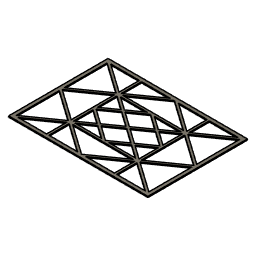
platform v3 (Autodesk Fusion 360 design; units mm, degrees)
Autodesk Fusion 360 part; units mm, degrees
sketch "Sketch1" plane through (0, 0, 0) normal (0, 1, 0) x (1, 0, 0)
  line L0 (178.39, 125.95) -> (-178.39, 125.95)
  line L1 (-178.39, 125.95) -> (-178.39, -125.95)
  line L2 (-178.39, -125.95) -> (178.39, -125.95)
  line L3 (178.39, -125.95) -> (178.39, 125.95)
  line L4 (178.39, 125.95) -> (-178.39, -125.95) construction
  line L5 (-178.39, 125.95) -> (178.39, -125.95) construction
  line L6 (-178.39, 0) -> (0, 125.95) construction
  line L7 (0, 125.95) -> (178.39, 0) construction
  line L8 (178.39, 0) -> (0, -125.95) construction
  line L9 (-178.39, 0) -> (0, -125.95) construction
  line L10 (-89.195, -62.975) -> (89.195, -62.975) construction
  line L11 (-89.195, 62.975) -> (89.195, 62.975) construction
  line L12 (89.195, 62.975) -> (89.195, -62.975) construction
  line L13 (-89.195, -62.975) -> (-89.195, 62.975) construction
  line L14 (-89.195, 0) -> (0, 62.975) construction
  line L15 (0, 62.975) -> (89.195, 0) construction
  line L16 (89.195, 0) -> (0, -62.975) construction
  line L17 (-89.195, 0) -> (0, -62.975) construction
  line L18 (-89.195, -62.975) -> (-89.195, -125.95) construction
  line L19 (89.195, -62.975) -> (89.195, -125.95) construction
  line L20 (89.195, 62.975) -> (89.195, 125.95) construction
  line L21 (-89.195, 62.975) -> (-89.195, 125.95) construction
  line L22 (-178.39, 125.95) -> (-89.195, 62.975)
  line L23 (-89.195, 62.975) -> (-90.9253, 60.5243)
  line L24 (-90.9253, 60.5243) -> (-180.1203, 123.4993)
  line L25 (-180.1203, 123.4993) -> (-178.39, 125.95)
  line L26 (-87.4647, 65.4257) -> (-176.6597, 128.4007)
  line L27 (-89.195, 62.975) -> (-87.4647, 65.4257)
  line L28 (-176.6597, 128.4007) -> (-178.39, 125.95)
  line L29 (-89.195, 125.95) -> (-89.195, 62.975)
  line L30 (-89.195, 62.975) -> (-92.195, 62.975)
  line L31 (-92.195, 62.975) -> (-92.195, 125.95)
  line L32 (-92.195, 125.95) -> (-89.195, 125.95)
  line L33 (-86.195, 62.975) -> (-86.195, 125.95)
  line L34 (-89.195, 62.975) -> (-86.195, 62.975)
  line L35 (-178.39, 0) -> (-89.195, 62.975)
  line L36 (-89.195, 62.975) -> (-90.9253, 65.4257)
  line L37 (-90.9253, 65.4257) -> (-180.1203, 2.4507)
  line L38 (-180.1203, 2.4507) -> (-178.39, 0)
  line L39 (-87.4647, 60.5243) -> (-176.6597, -2.4507)
  line L40 (-89.195, 62.975) -> (-87.4647, 60.5243)
  line L41 (-89.195, 62.975) -> (-89.195, 0)
  line L42 (-89.195, 0) -> (-92.195, 0)
  line L43 (-92.195, 0) -> (-92.195, 62.975)
  line L44 (-92.195, 62.975) -> (-89.195, 62.975)
  line L45 (-86.195, 0) -> (-86.195, 62.975)
  line L46 (-89.195, 0) -> (-86.195, 0)
  line L47 (-89.195, 0) -> (0, 62.975)
  line L48 (0, 62.975) -> (1.7303, 60.5243)
  line L49 (1.7303, 60.5243) -> (-87.4647, -2.4507)
  line L50 (-87.4647, -2.4507) -> (-89.195, 0)
  line L51 (0, 62.975) -> (-1.7303, 65.4257)
  line L52 (-1.7303, 65.4257) -> (-90.9253, 2.4507)
  line L53 (178.39, -125.95) -> (-89.195, 62.975)
  line L54 (-89.195, 62.975) -> (-87.4647, 65.4257)
  line L55 (-87.4647, 65.4257) -> (180.1203, -123.4993)
  line L56 (180.1203, -123.4993) -> (178.39, -125.95)
  line L57 (-90.9253, 60.5243) -> (176.6597, -128.4007)
  line L58 (0, 125.95) -> (-89.195, 62.975)
  line L59 (-89.195, 62.975) -> (-87.4647, 60.5243)
  line L60 (-87.4647, 60.5243) -> (1.7303, 123.4993)
  line L61 (1.7303, 123.4993) -> (0, 125.95)
  line L62 (-90.9253, 65.4257) -> (-1.7303, 128.4007)
  line L63 (-89.195, 62.975) -> (89.195, 62.975)
  line L64 (89.195, 62.975) -> (89.195, 65.975)
  line L65 (89.195, 65.975) -> (-89.195, 65.975)
  line L66 (-89.195, 65.975) -> (-89.195, 62.975)
  line L67 (89.195, 59.975) -> (-89.195, 59.975)
  line L68 (0, 62.975) -> (89.195, 0)
  line L69 (89.195, 0) -> (90.9253, 2.4507)
  line L70 (90.9253, 2.4507) -> (1.7303, 65.4257)
  line L71 (1.7303, 65.4257) -> (0, 62.975)
  line L72 (87.4647, -2.4507) -> (-1.7303, 60.5243)
  line L73 (-178.39, -125.95) -> (178.39, 125.95)
  line L74 (178.39, 125.95) -> (176.6597, 128.4007)
  line L75 (176.6597, 128.4007) -> (-180.1203, -123.4993)
  line L76 (-180.1203, -123.4993) -> (-178.39, -125.95)
  line L77 (180.1203, 123.4993) -> (-176.6597, -128.4007)
  line L78 (-89.195, -125.95) -> (-89.195, 0)
  line L79 (-89.195, 0) -> (-92.195, 0)
  line L80 (-92.195, 0) -> (-92.195, -125.95)
  line L81 (-92.195, -125.95) -> (-89.195, -125.95)
  line L82 (-86.195, 0) -> (-86.195, -125.95)
  line L83 (-178.39, 0) -> (0, -125.95)
  line L84 (0, -125.95) -> (1.7303, -123.4993)
  line L85 (1.7303, -123.4993) -> (-176.6597, 2.4507)
  line L86 (-176.6597, 2.4507) -> (-178.39, 0)
  line L87 (-1.7303, -128.4007) -> (-180.1203, -2.4507)
  line L88 (0, -62.975) -> (-89.195, 0)
  line L89 (-89.195, 0) -> (-87.4647, 2.4507)
  line L90 (-87.4647, 2.4507) -> (1.7303, -60.5243)
  line L91 (1.7303, -60.5243) -> (0, -62.975)
  line L92 (-90.9253, -2.4507) -> (-1.7303, -65.4257)
  line L93 (178.39, 0) -> (0, -125.95)
  line L94 (0, -125.95) -> (-1.7303, -123.4993)
  line L95 (-1.7303, -123.4993) -> (176.6597, 2.4507)
  line L96 (176.6597, 2.4507) -> (178.39, 0)
  line L97 (1.7303, -128.4007) -> (180.1203, -2.4507)
  line L98 (0, 125.95) -> (178.39, 0)
  line L99 (178.39, 0) -> (180.1203, 2.4507)
  line L100 (180.1203, 2.4507) -> (1.7303, 128.4007)
  line L101 (1.7303, 128.4007) -> (0, 125.95)
  line L102 (176.6597, -2.4507) -> (-1.7303, 123.4993)
  line L103 (89.195, 125.95) -> (89.195, -125.95)
  line L104 (89.195, -125.95) -> (92.195, -125.95)
  line L105 (92.195, -125.95) -> (92.195, 125.95)
  line L106 (92.195, 125.95) -> (89.195, 125.95)
  line L107 (86.195, -125.95) -> (86.195, 125.95)
  line L108 (0, -62.975) -> (89.195, 0)
  line L109 (89.195, 0) -> (87.4647, 2.4507)
  line L110 (87.4647, 2.4507) -> (-1.7303, -60.5243)
  line L111 (-1.7303, -60.5243) -> (0, -62.975)
  line L112 (90.9253, -2.4507) -> (1.7303, -65.4257)
  line L113 (-89.195, -62.975) -> (89.195, -62.975)
  line L114 (89.195, -62.975) -> (89.195, -59.975)
  line L115 (89.195, -59.975) -> (-89.195, -59.975)
  line L116 (-89.195, -59.975) -> (-89.195, -62.975)
  line L117 (89.195, -65.975) -> (-89.195, -65.975)
  line L118 (-178.39, 125.95) -> (-174.39, 125.95)
  line L119 (-174.39, 125.95) -> (-174.39, -126.4932)
  line L120 (-174.39, -126.4932) -> (-178.39, -126.4932)
  line L121 (-178.39, -126.4932) -> (-178.39, 125.95)
  line L122 (-178.39, -125.95) -> (178.39, -125.95)
  line L123 (178.39, -125.95) -> (178.39, -121.95)
  line L124 (178.39, -121.95) -> (-178.39, -121.95)
  line L125 (-178.39, -121.95) -> (-178.39, -125.95)
  line L126 (178.39, 125.95) -> (174.39, 125.95)
  line L127 (174.39, 125.95) -> (174.39, -125.95)
  line L128 (174.39, -125.95) -> (178.39, -125.95)
  line L129 (178.39, -125.95) -> (178.39, 125.95)
  line L130 (178.39, 125.95) -> (-178.39, 125.95)
  line L131 (-178.39, 125.95) -> (-178.39, 121.95)
  line L132 (-178.39, 121.95) -> (178.39, 121.95)
  line L133 (178.39, 121.95) -> (178.39, 125.95)
  line L134 (183.39, 130.95) -> (-183.39, 130.95)
  line L135 (-183.39, 130.95) -> (-183.39, -130.95)
  line L136 (-183.39, -130.95) -> (183.39, -130.95)
  line L137 (183.39, -130.95) -> (183.39, 130.95)
  line L138 (183.39, 130.95) -> (-183.39, -130.95) construction
  line L139 (-183.39, 130.95) -> (183.39, -130.95) construction
  line L140 (0, 130.95) -> (0, 125.95) construction
  line L141 (-183.39, 66.313) -> (-178.39, 66.313) construction
  dimension "d1" = 356.78
  dimension "d2" = 251.9
  dimension "d3" = 3
  dimension "d4" = 3
  dimension "d5" = 3
  dimension "d6" = 3
  dimension "d7" = 3
  dimension "d8" = 3
  dimension "d9" = 3
  dimension "d10" = 3
  dimension "d11" = 3
  dimension "d12" = 3
  dimension "d13" = 3
  dimension "d14" = 3
  dimension "d15" = 3
  dimension "d16" = 3
  dimension "d17" = 3
  dimension "d18" = 3
  dimension "d19" = 3
  dimension "d20" = 3
  dimension "d21" = 4
  dimension "d22" = 4
  dimension "d23" = 4
  dimension "d24" = 4
  dimension "d27" = 5
  constraint horizontal L0
  constraint perpendicular L0 L1
  constraint parallel L0 L2
  constraint parallel L1 L3
  constraint coincident L4 origin
  constraint coincident L5 origin
  constraint midpoint L1 L6.start
  constraint midpoint L0 L6.end
  constraint midpoint L3 L7.end
  constraint midpoint L2 L8.end
  constraint midpoint L9 L10.start
  constraint midpoint L8 L10.end
  constraint midpoint L6 L11.start
  constraint midpoint L7 L11.end
  constraint midpoint L13 L14.start
  constraint midpoint L11 L14.end
  constraint midpoint L12 L15.end
  constraint midpoint L10 L16.end
  constraint coincident L2 L18.end
  constraint perpendicular L2 L18
  constraint coincident L2 L19.end
  constraint perpendicular L2 L19
  constraint coincident L0 L20.end
  constraint perpendicular L0 L20
  constraint coincident L0 L21.end
  constraint perpendicular L0 L21
  constraint perpendicular L22 L23
  constraint parallel L22 L24
  constraint parallel L23 L25
  constraint symmetric L0.end L5 L1.start
  constraint symmetric L5 L11.start L13.end
  constraint symmetric L5 L23.end L26.start
  constraint symmetric L5 L24.end L26.end
  constraint perpendicular L29 L30
  constraint parallel L29 L31
  constraint parallel L30 L32
  constraint symmetric L21 L11.start L13.end
  constraint symmetric L21 L30.end L33.start
  constraint symmetric L21 L31.end L33.end
  constraint perpendicular L35 L36
  constraint parallel L35 L37
  constraint parallel L36 L38
  constraint symmetric L6 L11.start L13.end
  constraint symmetric L6 L36.end L39.start
  constraint symmetric L6 L37.end L39.end
  constraint perpendicular L41 L42
  constraint parallel L41 L43
  constraint parallel L42 L44
  constraint symmetric L14.start L41 L17.start
  constraint symmetric L42.end L41 L45.start
  constraint symmetric L30.end L41 L33.start
  constraint perpendicular L47 L48
  constraint parallel L47 L49
  constraint parallel L48 L50
  constraint symmetric L15.start L14 L47.end
  constraint symmetric L14 L48.end L51.end
  constraint symmetric L14 L49.end L52.end
  constraint perpendicular L53 L54
  constraint parallel L53 L55
  constraint parallel L54 L56
  constraint symmetric L26.start L53 L23.end
  constraint symmetric L55.end L53 L57.end
  constraint perpendicular L58 L59
  constraint parallel L58 L60
  constraint parallel L59 L61
  constraint symmetric L39.start L58 L36.end
  constraint symmetric L60.end L58 L62.end
  constraint perpendicular L63 L64
  constraint parallel L63 L65
  constraint parallel L64 L66
  constraint symmetric L64.end L63 L67.start
  constraint symmetric L65.end L63 L67.end
  constraint perpendicular L68 L69
  constraint parallel L68 L70
  constraint parallel L69 L71
  constraint symmetric L15 L69.end L72.start
  constraint symmetric L15 L70.end L72.end
  constraint perpendicular L73 L74
  constraint parallel L73 L75
  constraint parallel L74 L76
  constraint symmetric L4 L74.end L77.start
  constraint symmetric L4 L75.end L77.end
  constraint perpendicular L78 L79
  constraint parallel L78 L80
  constraint parallel L79 L81
  constraint symmetric L13 L42.end L45.start
  constraint symmetric L13 L80.end L82.end
  constraint perpendicular L83 L84
  constraint parallel L83 L85
  constraint parallel L84 L86
  constraint symmetric L9 L84.end L87.start
  constraint symmetric L9 L85.end L87.end
  constraint perpendicular L88 L89
  constraint parallel L88 L90
  constraint parallel L89 L91
  constraint symmetric L89.end L88 L92.start
  constraint symmetric L90.end L88 L92.end
  constraint perpendicular L93 L94
  constraint parallel L93 L95
  constraint parallel L94 L96
  constraint symmetric L8 L94.end L97.start
  constraint symmetric L8 L95.end L97.end
  constraint perpendicular L98 L99
  constraint parallel L98 L100
  constraint parallel L99 L101
  constraint symmetric L99.end L98 L102.start
  constraint symmetric L100.end L98 L102.end
  constraint perpendicular L103 L104
  constraint parallel L103 L105
  constraint parallel L104 L106
  constraint symmetric L19 L104.end L107.start
  constraint symmetric L19 L105.end L107.end
  constraint perpendicular L108 L109
  constraint parallel L108 L110
  constraint parallel L109 L111
  constraint symmetric L16 L109.end L112.start
  constraint symmetric L16 L110.end L112.end
  constraint perpendicular L113 L114
  constraint parallel L113 L115
  constraint parallel L114 L116
  constraint symmetric L10 L114.end L117.start
  constraint symmetric L10 L115.end L117.end
  constraint horizontal L118
  constraint vertical L119
  constraint horizontal L120
  constraint vertical L121
  constraint horizontal L122
  constraint vertical L123
  constraint horizontal L124
  constraint vertical L125
  constraint horizontal L126
  constraint vertical L127
  constraint horizontal L128
  constraint vertical L129
  constraint coincident L122 L127.end
  constraint horizontal L130
  constraint vertical L131
  constraint horizontal L132
  constraint vertical L133
  constraint horizontal L134
  constraint perpendicular L134 L135
  constraint parallel L134 L136
  constraint parallel L135 L137
  constraint coincident L138 origin
  constraint coincident L139 origin
  constraint midpoint L134 L140.start
  constraint coincident L135 L141.start
  constraint coincident L121 L141.end
  constraint perpendicular L121 L141
  constraint equal L140 L141
  measures "d1" distance of L0.start L0.end
  measures "d2" distance of L0.start L2.end
  measures "d3" distance of L0.end L24.end
  measures "d4" distance of L21.end L31.end
  measures "d5" distance of L6.start L37.end
  measures "d6" distance of L11.start L30.end
  measures "d7" distance of L14.start L49.end
  measures "d8" distance of L2.end L55.end
  measures "d9" distance of L6.end L60.end
  measures "d10" distance of L11.start L65.end
  measures "d11" distance of L14.end L70.end
  measures "d12" distance of L1.end L75.end
  measures "d13" distance of L18.end L80.end
  measures "d14" distance of L6.start L85.end
  measures "d15" distance of L16.end L90.end
  measures "d16" distance of L7.end L95.end
  measures "d17" distance of L6.end L100.end
  measures "d18" distance of L20.end L105.end
  measures "d19" distance of L16.end L110.end
  measures "d20" distance of L10.start L115.end
  measures "d21" distance of L0.end L118.end
  measures "d22" distance of L1.end L124.end
  measures "d23" distance of L0.start L126.end
  measures "d24" distance of L0.start L132.end
  measures "d27" distance of L141.start L141.end
extrude "Extrude1" add sketch "Sketch1" along normal blind 2.75 contours L0 L73 L126 L127 L130 | L3 L73 L77 L127 L129 L132 L133 | L0 L74 L75 L126 L130 | L0 L73 L75 L127 L130 L132 | L3 L77 L129 L132 L133 | L73 L127 L132 | L0 L75 L105 L130 L132 | L3 L77 L100 L127 L129 L132 | L77 L127 L132 | L73 L77 L100 L105 L127 L132 | L73 L75 L105 L132 | L0 L103 L105 L106 L130 L132 | L3 L99 L100 L129 | L3 L95 L96 L98 L100 L127 L129 | L73 L100 L105 | L73 L75 L100 L105 | L0 L103 L107 L130 L132 | L75 L103 L105 L132 | L3 L93 L97 L127 L129 | L95 L96 L98 | L93 L95 L98 L102 L127 | L77 L98 L100 L105 L127 | L77 L100 L105 | L73 L77 L98 L100 L105 | L64 L73 L100 L103 | L0 L100 L107 L130 L132 | L100 L103 L107 L132 | L65 L75 L103 | L65 L75 L100 L107 | L3 L55 L97 L124 L127 L129 | L93 L102 L127 | L95 L98 L127 | L95 L98 L102 L105 L127 | L77 L98 L105 | L63 L73 L102 L107 | L64 L65 L75 L98 L103 | L67 L73 L102 L103 | L63 L75 L98 L107 | L77 L98 L103 | L0 L98 L100 L130 L132 | L0 L100 L101 L130 | L65 L75 L98 L107 | L65 L98 L100 L107 L132 | L3 L55 L123 L124 L129 | L55 L93 L97 L105 L127 | L93 L95 L102 L105 L127 | L95 L102 L127 | L77 L98 L102 L105 | L63 L102 L107 | L63 L75 L107 | L67 L73 L102 L107 | L73 L102 L107 | L75 L98 L107 | L67 L102 L103 | L0 L58 L62 L130 L132 | L58 L60 L61 L132 | L60 L61 L98 L102 L132 | L65 L98 L107 | L3 L55 L56 L123 L129 | L3 L53 L55 L123 L124 L127 L129 | L55 L124 L127 | L55 L97 L105 | L53 L55 L97 L105 L124 L127 | L55 L93 L105 | L55 L93 L95 L105 | L69 L70 L95 L102 L103 L105 | L70 L77 L103 L107 | L67 L77 L102 L107 | L63 L67 L70 L75 | L65 L75 L98 L102 L107 | L67 L73 L75 L102 L107 | L51 L52 L60 L63 L65 L70 L71 L102 | L67 L73 L107 | L0 L33 L62 L130 L132 | L58 L60 L65 L132 | L33 L58 L62 L65 L132 | L65 L98 L102 L132 | L2 L53 L122 L127 L128 | L53 L124 L127 | L53 L55 L93 L97 L105 | L53 L97 L105 | L55 L93 L103 L114 | L67 L70 L73 L77 L107 | L68 L70 L103 L107 L109 L110 | L69 L70 L103 | L63 L67 L68 L70 | L63 L70 L71 | L67 L70 L73 L75 | L0 L29 L33 L130 L132 | L33 L55 L58 L60 L65 | L33 L58 L65 | L60 L102 L132 | L2 L53 L57 L122 L124 L127 | L53 L57 L105 L124 | L53 L97 L103 | L53 L57 L97 L105 | L55 L95 L107 L115 | L95 L103 L115 | L55 L103 L107 L112 | L53 L95 L107 L113 | L57 L93 L103 L117 | L53 L95 L103 L114 L115 | L57 L93 L107 L113 | L68 L70 L73 L77 | L68 L70 L77 L107 | L68 L72 L107 L108 L110 | L103 L107 L108 L112 | L68 L109 L110 | L47 L48 L49 L67 | L48 L49 L67 L68 | L51 L52 L63 | L47 L52 L63 L67 | L67 L68 L70 L75 | L68 L70 L73 L75 | L0 L29 L31 L32 L130 L132 | L29 L33 L62 L132 | L26 L33 L62 L65 | L26 L33 L55 L58 L65 | L33 L55 L58 | L2 L57 L105 L122 L124 | L57 L97 L107 L117 | L97 L103 L107 L124 | L57 L103 L117 | L57 L103 L105 L124 | L53 L55 L107 L112 L115 | L53 L95 L107 L115 | L53 L95 L107 | L57 L93 L107 | L57 L93 L107 L117 | L95 L107 L113 | L57 L107 L113 | L68 L72 L73 L77 | L68 L72 L77 L107 L110 | L68 L107 L110 | L72 L107 L108 | L47 L49 L55 L67 L72 | L47 L52 L55 L67 | L52 L55 L63 L67 | L49 L67 L68 L72 L75 | L68 L72 L73 L75 | L33 L55 L63 | L45 L53 L55 L60 L67 | L45 L60 L63 | L0 L26 L31 L130 L132 | L26 L29 L31 L132 | L22 L26 L31 L37 L62 | L26 L29 L65 | L29 L36 L62 L66 | L33 L34 L55 L58 L63 | L27 L54 L55 L58 | L26 L27 L29 L54 L65 L66 | L2 L103 L104 L105 L122 L124 | L93 L97 L107 L117 L124 | L2 L103 L107 L122 L124 | L53 L55 L108 L112 | L55 L107 L108 L112 | L53 L107 L115 | L53 L57 L95 L107 L115 | L57 L93 L95 L107 L117 | L93 L107 L117 | L57 L112 L113 L115 | L85 L95 L113 L117 | L55 L72 L73 L77 | L72 L107 L110 | L55 L72 L107 L108 L110 | L47 L49 L53 L55 | L47 L52 L53 L55 | L49 L67 L72 | L55 L72 L73 L75 | L52 L53 L55 L67 | L34 L45 L53 L60 L63 | L45 L53 L60 | L0 L22 L26 L119 L130 L132 | L0 L26 L28 L118 L130 | L22 L26 L31 L132 | L22 L36 L37 | L22 L30 L31 L37 L44 | L23 L41 L57 | L24 L30 L35 L43 L44 | L23 L24 L35 | L40 L53 L59 L60 | L39 L40 L41 L59 L67 | L2 L97 L107 L122 L124 | L2 L93 L97 L122 L124 | L53 L55 L108 L110 | L53 L57 L108 L112 | L53 L57 L112 L115 | L93 L95 L117 L124 | L108 L112 L113 L115 | L53 L55 L73 L77 | L53 L55 L77 L110 | L47 L49 L53 L57 | L47 L52 L53 L57 | L49 L53 L55 L75 | L53 L55 L73 L75 | L45 L53 L67 | L45 L52 L53 L57 L67 | L39 L45 L53 L60 L67 | L0 L22 L118 L119 L130 | L22 L24 L31 L37 L119 L132 | L22 L31 L37 | L24 L35 L39 L43 L57 | L24 L31 L37 L43 | L24 L35 L43 | L39 L41 L67 | L84 L85 L93 L95 L124 | L53 L57 L108 L110 | L57 L108 L112 L115 | L85 L95 L124 | L77 L82 L83 L85 L117 | L83 L85 L117 L124 | L88 L92 L113 L115 | L90 L91 L110 L111 L115 | L90 L91 L108 L115 | L88 L110 L111 L115 | L53 L57 L73 L77 | L53 L57 L77 L110 | L45 L47 L49 L57 L90 | L45 L47 L52 L57 | L49 L53 L57 L75 | L53 L57 L73 L75 | L39 L45 L57 L67 | L1 L22 L24 L119 L121 L131 L132 | L1 L24 L25 L121 L131 | L22 L119 L132 | L39 L41 L42 L43 L79 | L41 L45 L52 L57 | L24 L35 L37 L43 L119 | L35 L39 L43 L85 L119 | L2 L83 L87 L122 L124 | L84 L85 L94 L95 | L83 L85 L94 L95 L124 | L57 L90 L108 L110 L115 | L73 L77 L82 L85 L115 | L82 L85 L113 | L77 L82 L113 | L77 L92 L113 L115 | L82 L83 L117 | L82 L83 L87 L117 L124 | L77 L88 L92 L115 | L77 L88 L90 L110 L115 | L57 L73 L77 L90 | L41 L45 L47 L52 L89 L90 | L45 L47 L90 | L57 L73 L75 L90 | L1 L24 L121 L131 L132 | L24 L119 L132 | L35 L85 L119 | L1 L35 L37 L85 L86 L119 L121 | L2 L82 L87 L122 L124 | L90 L110 L115 | L73 L77 L92 L115 | L77 L82 L83 | L77 L82 L83 L113 | L73 L82 L85 | L73 L82 L85 L113 | L77 L82 L83 L117 | L77 L82 L87 L117 | L73 L77 L88 L90 | L73 L77 L88 L92 | L45 L49 L82 L90 | L45 L46 L47 L90 | L47 L89 L90 | L49 L75 L82 L88 L90 | L73 L75 L88 L90 | L1 L24 L37 L119 L121 L132 | L39 L80 L83 L85 L119 | L39 L85 L119 | L42 L78 L79 L80 L85 | L49 L50 L88 | L49 L50 L78 L82 L88 L92 | L46 L49 L82 L88 | L35 L39 L83 L85 L119 | L35 L85 L86 | L2 L78 L82 L122 L124 | L73 L75 L82 L92 L115 | L73 L82 L115 | L77 L78 L83 L117 | L73 L82 L85 L115 | L73 L78 L85 L115 L116 | L73 L78 L87 | L75 L78 L83 L116 | L73 L75 L80 L83 L87 | L78 L82 L87 L124 | L77 L78 L117 | L73 L75 L88 L92 | L49 L82 L88 | L75 L82 L88 L92 | L1 L37 L38 L121 | L39 L83 L119 | L75 L80 L83 L85 | L75 L78 L82 L92 | L1 L83 L87 L119 L121 | L2 L78 L80 L81 L122 L124 | L75 L82 L85 L115 | L78 L85 L115 | L73 L77 L80 L87 | L73 L80 L87 | L75 L80 L83 | L77 L78 L80 L124 | L75 L80 L83 L87 L119 | L1 L75 L87 L119 L121 L124 | L2 L77 L80 L122 L124 | L73 L77 L80 L124 | L73 L75 L80 L87 L119 L124 | L75 L80 L87 | L1 L75 L121 L124 L125 | L2 L73 L77 L119 L122 L124 | L73 L119 L124 | L75 L119 L124 | L1 L73 L75 L119 L121 L124 L125 | L1 L75 L76 L121 L125 | L2 L119 L120 L121 L122 | L2 L73 L119 L122 | L134 L135 L136 L137
